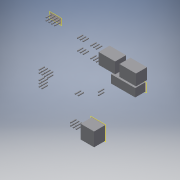
# Autodesk Inventor part: connectors
Saved by Autodesk Inventor 2016 (Build 200138000, 138)
## iProperties
Created: 2016-03-25
Part Number: connectors
Material: Generic
Document SubType Name: Sheet Metal
Designer: Paschalis
Density: 1 g/cm^3
Sheet Metal Rule: Default
Appearance: Default
Author: Paschalis
Autodesk Inventor part; units mm, degrees
ref_plane "YZ Plane" through (0, 0, 0) normal (1, 0, 0) x (0, 1, 0)
ref_plane "XZ Plane" through (0, 0, 0) normal (0, 1, 0) x (-1, 0, 0)
ref_plane "XY Plane" through (0, 0, 0) normal (0, 0, 1) x (1, 0, 0)
sketch "Sketch1" plane through (0, 0, 0) normal (0, 0, 1) x (1, 0, 0)
  line L0 (7.5318, 5.0635) -> (-7.5317, 5.0635) projected
  line L1 (-7.5317, 5.0635) -> (-7.5317, -5.0635) projected
  line L2 (-7.5317, -5.0635) -> (7.5317, -5.0635) projected
  line L3 (7.5317, -5.0635) -> (7.5318, 5.0635) projected
  line L4 (11.4548, -5.0635) -> (26.5183, -5.0635) projected
  line L5 (26.5183, -5.0635) -> (26.5182, 5.0635) projected
  line L6 (26.5182, 5.0635) -> (11.4547, 5.0635) projected
  line L7 (11.4547, 5.0635) -> (11.4548, -5.0635) projected
  point P0 (0, 0)
extrude "Extrusion1" add sketch "Sketch1" along normal blind 10
ref_plane "Work Plane1" through (-17.761, -65.8967, 0) normal (0, 0, 1) x (-1, 0, 0)
sketch "Sketch2" plane through (-17.761, -65.8967, 0) normal (0, 0, 1) x (-1, 0, 0)
  line L0 (6.1468, 6.2068) -> (-6.1468, 6.2068) projected
  line L1 (-6.1468, 6.2068) -> (-6.1468, -6.2067) projected
  line L2 (-6.1468, -6.2067) -> (6.1468, -6.2067) projected
  line L3 (6.1468, -6.2067) -> (6.1468, 6.2068) projected
  point P0 (-17.761, -65.8967)
extrude "Extrusion2" add sketch "Sketch2" along normal blind 10
ref_plane "Work Plane2" through (-56.5087, 1.9431, 0) normal (0, 0, 1) x (-1, 0, 0)
sketch "Sketch3" plane through (-56.5087, 1.9431, 0) normal (0, 0, 1) x (-1, 0, 0)
  circle A0 centre (3.8531, -1.2269) radius 0.51 projected
  circle A1 centre (1.3031, -1.2269) radius 0.51 projected
  circle A2 centre (-1.2369, -1.2269) radius 0.51 projected
  circle A3 centre (-3.7669, -1.2269) radius 0.51 projected
  circle A4 centre (-3.7669, 1.3031) radius 0.51 projected
  circle A5 centre (-1.2369, 1.3031) radius 0.51 projected
  circle A6 centre (1.3031, 1.3031) radius 0.51 projected
  circle A7 centre (3.8531, 1.3031) radius 0.51 projected
  circle A8 centre (2.5731, 43.2131) radius 0.51 projected
  circle A9 centre (2.5731, 45.7531) radius 0.51 projected
  circle A10 centre (5.1131, 45.7531) radius 0.51 projected
  circle A11 centre (5.1131, 43.2131) radius 0.51 projected
  circle A12 centre (7.6531, 43.2131) radius 0.51 projected
  circle A13 centre (7.6531, 45.7531) radius 0.51 projected
  line L0 (1.3081, 41.9481) -> (11.5443, 41.9481) projected
  line L1 (11.5443, 41.9481) -> (11.5443, 47.1043) projected
  line L2 (11.5443, 47.1043) -> (1.3081, 47.1043) projected
  line L3 (1.3081, 47.1043) -> (1.3081, 41.9481) projected
  circle A14 centre (10.1931, 43.2131) radius 0.51 projected
  circle A15 centre (10.1931, 45.7531) radius 0.51 projected
  line L4 (11.5443, 47.1043) -> (1.3081, 47.1043) projected
  line L5 (11.5443, 41.9481) -> (11.5443, 47.1043) projected
  circle A16 centre (7.6531, 51.4731) radius 0.51 projected
  line L6 (11.4681, 50.2031) -> (11.4681, 57.9247) projected
  line L7 (11.4681, 57.9247) -> (6.0531, 57.9247) projected
  line L8 (6.0531, 57.9247) -> (6.0531, 50.2031) projected
  line L9 (6.0531, 50.2031) -> (11.4681, 50.2031) projected
  circle A17 centre (10.1931, 51.4731) radius 0.51 projected
  circle A18 centre (10.1931, 54.0131) radius 0.51 projected
  circle A19 centre (7.6531, 54.0131) radius 0.51 projected
  circle A20 centre (7.6531, 56.5531) radius 0.51 projected
  circle A21 centre (10.1931, 56.5531) radius 0.51 projected
  circle A22 centre (-23.4569, 73.0631) radius 0.55 projected
  circle A23 centre (-20.9169, 73.0631) radius 0.55 projected
  circle A24 centre (-18.3769, 73.0631) radius 0.55 projected
  circle A25 centre (-18.3769, 70.5231) radius 0.55 projected
  circle A26 centre (-20.9169, 70.5231) radius 0.55 projected
  line L10 (-25.0204, 67.3596) -> (-16.8134, 67.3596) projected
  line L11 (-16.8134, 67.3596) -> (-16.8134, 74.0631) projected
  line L12 (-16.8134, 74.0631) -> (-25.0204, 74.0631) projected
  line L13 (-25.0204, 74.0631) -> (-25.0204, 67.3596) projected
  circle A27 centre (-23.4569, 70.5231) radius 0.55 projected
  circle A28 centre (-22.7469, 45.6731) radius 0.51 projected
  circle A29 centre (-25.2869, 45.6731) radius 0.51 projected
  circle A30 centre (-43.7769, 36.2331) radius 0.51 projected
  circle A31 centre (-43.7769, 33.6931) radius 0.51 projected
  circle A32 centre (-24.7269, 0.6731) radius 0.51 projected
  circle A33 centre (-27.2669, 0.6731) radius 0.51 projected
  circle A34 centre (-29.8069, 0.6731) radius 0.51 projected
  circle A35 centre (-36.7969, 0.6731) radius 0.51 projected
  circle A36 centre (-39.3369, 0.6731) radius 0.51 projected
  circle A37 centre (-41.8769, 0.6731) radius 0.51 projected
  circle A38 centre (-41.8769, 10.8331) radius 0.51 projected
  circle A39 centre (-39.3369, 10.8331) radius 0.51 projected
  circle A40 centre (-36.7969, 10.8331) radius 0.51 projected
  circle A41 centre (-29.8069, 10.8331) radius 0.51 projected
  circle A42 centre (-27.2669, 10.8331) radius 0.51 projected
  circle A43 centre (-24.7269, 10.8331) radius 0.51 projected
  point P0 (-56.5086, 1.9431)
extrude "Extrusion3" add sketch "Sketch3" along normal blind 5 contours A0 | A1 | A2 | A3 | A4 | A5 | A6 | A7 | A8 | A9 | A10 | A11 | A12 | A13 | A14 | A15 | A16 | A17 | A18 | A19 | A20 | A21 | A22 | A23 | A24 | A25 | A26 | A27 | A28 | A29 | A30 | A31 | A32 | A33 | A34 | A35 | A36 | A37 | A38 | A39 | A40 | A41 | A42 | A43
ref_plane "Work Plane3" through (13.7793, -11.43, 0) normal (0, 0, 1) x (-1, 0, 0)
sketch "Sketch4" plane through (13.7793, -11.43, 0) normal (0, 0, 1) x (-1, 0, 0)
  line L0 (11.049, 3.683) -> (-11.049, 3.683) projected
  line L1 (-11.049, 3.683) -> (-11.049, -3.683) projected
  line L2 (-11.049, -3.683) -> (11.049, -3.683) projected
  line L3 (11.049, -3.683) -> (11.049, 3.683) projected
  point P0 (13.7792, -11.43)
extrude "Extrusion4" add sketch "Sketch4" along normal blind 9
equation "\"BendRadius\" = Thickness"
equation "\"BendReliefWidth\" = Thickness"
equation "\"BendReliefDepth\" = 0.5 * Thickness"
equation "\"CornerReliefSize\" = 4 * Thickness"
equation "\"MinimumRemnant\" = 2 * Thickness"
equation "\"TransitionRadius\" = BendRadius"
equation "\"JacobiRadiusSize\" = BendRadius"
equation "\"GapSize\" = Thickness"
equation "\"Thickness\" = 3.048"
body "Solid1"
